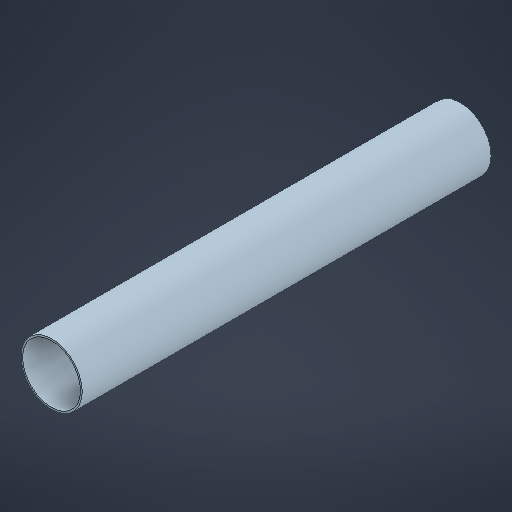
# Autodesk Inventor part: Probe_Tube
Saved by Autodesk Inventor 2027.1 (Build 311270010, 270A)
## iProperties
Created: 2026-09-21
Part Number: Probe_Tube
Material: Generic
Document SubType Name: Modeling
Designer: 박정현
Density: 1 g/cm^3
Appearance: Sleeve - material unspecified
Author: 박정현
Comments: Open-ended tube, ID 51 mm, OD 54 mm, length 360 mm. Part local axis is Z. In assembly the axis is Y through X=25.5 mm, Z=3 mm, the midpoint of the H-frame rod centre lines. Length matches rods by assumption. Requested dimensions retained even where existing geometry intersects.
Autodesk Inventor part; units mm, degrees
ref_plane "YZ Plane" through (0, 0, 0) normal (1, 0, 0) x (0, 1, 0)
ref_plane "XZ Plane" through (0, 0, 0) normal (0, 1, 0) x (-1, 0, 0)
ref_plane "XY Plane" through (0, 0, 0) normal (0, 0, 1) x (1, 0, 0)
sketch "Concentric_Tube_Section" plane through (0, 0, 0) normal (0, 0, 1) x (1, 0, 0)
  circle A0 centre (0, 0) radius 27
  circle A1 centre (0, 0) radius 25.5
  dimension "d0" = 54
  dimension "d1" = 51
  constraints: 2 centre point, 2 coincident
  measures "d0" diameter of A0
  measures "d1" diameter of A1
extrude "Open_Ended_Cylindrical_Sleeve" add sketch "Concentric_Tube_Section" along normal blind 360
equation "\"d0\" = OuterDiameter"
equation "\"d1\" = InnerDiameter"
equation "\"d2\" = TubeLength"
equation "\"InnerDiameter\" = 51"
equation "\"OuterDiameter\" = 54"
equation "\"TubeLength\" = 360"
equation "\"WallThickness\" = -0.5 * InnerDiameter + 0.5 * OuterDiameter"
body "Solid1"
